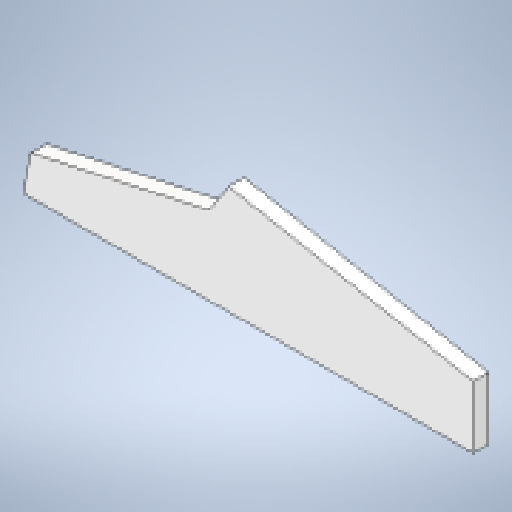
# Autodesk Inventor part: Side_Blocker
Saved by Autodesk Inventor 2023.2 (Build 272271000, 271)
## iProperties
Created: 2024-01-26
Part Number: Side_Blocker
Material: UHMW, White
Document SubType Name: Modeling
Designer: Nathan Cai
Mass: 17.3544 g
Surface Area: 114.912 cm^2
Volume: 18.4622 cm^3
Density: 0.94 g/cm^3
Appearance: Smooth - White
Author: Nathan Cai
Autodesk Inventor part; units mm, degrees
ref_plane "YZ Plane" through (0, 0, 0) normal (1, 0, 0) x (0, 1, 0)
ref_plane "XZ Plane" through (0, 0, 0) normal (0, 1, 0) x (-1, 0, 0)
ref_plane "XY Plane" through (0, 0, 0) normal (0, 0, 1) x (1, 0, 0)
sketch "Sketch1" plane through (0, 0, 0) normal (0, 0, 1) x (1, 0, 0)
  line L0 (0, 0) -> (184.15, 0)
  line L1 (84.0906, 44.45) -> (76.2, 32.0643)
  line L2 (76.2, 32.0643) -> (3.175, 15.875)
  line L3 (3.175, 15.875) -> (0, 0)
  circle A0 centre (0, 0) radius 190.5 construction
  line L4 (0, 0) -> (0, 190.5) construction
  line L5 (184.15, 0) -> (184.15, 25.4)
  line L6 (184.15, 25.4) -> (84.0906, 44.45)
  circle A1 centre (95.25, 12.7) radius 12
  dimension "d3" = 381
  dimension "d0" = 184.15
  dimension "d1" = 3.175
  dimension "d2" = 15.875
  dimension "d4" = 12.5
  dimension "d5" = 76.2
  dimension "d6" = 44.45
  dimension "d12" = 135
  dimension "d13" = 25.4
  dimension "d15" = 24
  dimension "d16" = 88.9
  dimension "d17" = 12.7
  constraints: 14 end point, 2 coincident, 2 vertical, 1 centre point, 1 perpendicular, 1 vertical alignment, 2 other
  measures "d0" distance of L0.start L0.end
  measures "d1" horizontal distance of point (0, 0) L2.end
  measures "d2" distance from line of L0 L2.end
  measures "d4" angle of L0 L2
  measures "d5" horizontal distance of point (0, 0) L1.end
  measures "d6" distance from line of L0 L1.start
  measures "d12" angle of L2 L1
  measures "d13" distance of L0.end L5.end
  measures "d15" diameter of A1
  measures "d16" distance from line of L5 A1.centre
  measures "d17" distance from line of L0 A1.centre
extrude "Extrusion1" add sketch "Sketch1" along normal blind 6.35 contours L3 L2 L1 L6 L5 L0 | A1
body "Solid1"
